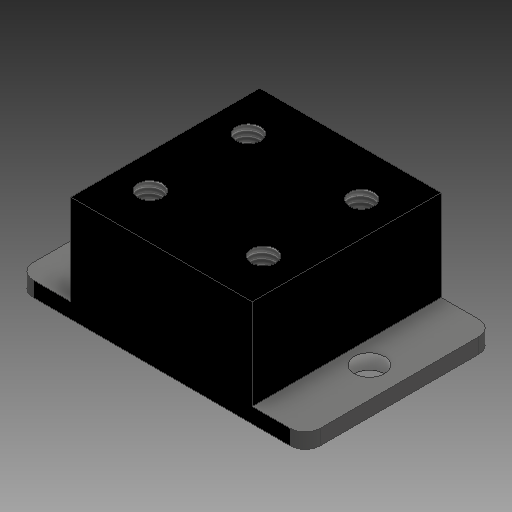
# Autodesk Inventor part: GT175DA120U
Saved by Autodesk Inventor 2019 (Build 230136000, 136)
## iProperties
Created: 2018-04-27
Part Number: GT175DA120U
Material: Generic
Document SubType Name: Modeling
Designer: Phil Erle
Density: 1 g/cm^3
Appearance: Default
Author: Phil Erle
Autodesk Inventor part; units mm, degrees
ref_plane "YZ Plane" through (0, 0, 0) normal (1, 0, 0) x (0, 1, 0)
ref_plane "XZ Plane" through (0, 0, 0) normal (0, 1, 0) x (-1, 0, 0)
ref_plane "XY Plane" through (0, 0, 0) normal (0, 0, 1) x (1, 0, 0)
sketch "Sketch1" plane through (0, 0, 0) normal (0, 0, 1) x (1, 0, 0)
  line L0 (-19, -12.5) -> (19, -12.5)
  line L1 (19, -12.5) -> (19, 12.5)
  line L2 (19, 12.5) -> (-19, 12.5)
  line L3 (-19, 12.5) -> (-19, -12.5)
  line L4 (-19, -12.5) -> (19, 12.5) construction
  line L5 (19, -12.5) -> (-19, 12.5) construction
  point P0 (0, 0)
  dimension "d0" = 38
  dimension "d1" = 25
  constraints: 12 end point, 2 midpoint, 2 parallel, 1 horizontal, 1 perpendicular
  measures "d0" distance of L1.end L2.end
  measures "d1" distance of L0.end L1.end
extrude "Extrusion1" add sketch "Sketch1" along normal blind 2
sketch "Sketch2" plane through (0, 0, 2) normal (0, 0, 1) x (1, 0, 0)
  line L0 (19, 12.5) -> (-19, 12.5) projected
  line L1 (-12, -12.5) -> (12, -12.5)
  line L2 (12, -12.5) -> (12, 12.5)
  line L3 (12, 12.5) -> (-12, 12.5)
  line L4 (-12, 12.5) -> (-12, -12.5)
  line L5 (-12, -12.5) -> (12, 12.5) construction
  line L6 (12, -12.5) -> (-12, 12.5) construction
  point P0 (0, 0)
  dimension "d4" = 24
  constraints: 12 end point, 2 midpoint, 2 parallel, 1 horizontal, 1 perpendicular, 1 point on line
  measures "d4" distance between parallel lines of L2 L4
extrude "Extrusion2" add sketch "Sketch2" along normal blind 12
sketch "Sketch3" plane through (0, 0, 2) normal (0, 0, 1) x (1, 0, 0)
  line L0 (-15, 0) -> (15, 0) construction
  point P0 (0, 0)
  point P1 (0, 0)
  dimension "d7" = 30
  constraints: 3 coincident, 2 end point, 1 horizontal, 1 horizontal alignment, 1 midpoint
  measures "d7" distance of L0.start L0.end
hole "Hole1" at (-15, 0, 2) at (15, 0, 2) direction (0, 0, -1) diameter 4 end through all
sketch "Sketch4" plane through (0, 0, 14) normal (0, 0, 1) x (1, 0, 0)
  line L0 (-7.5, -6.5) -> (7.5, -6.5) construction
  line L1 (7.5, -6.5) -> (7.5, 6.5) construction
  line L2 (7.5, 6.5) -> (-7.5, 6.5) construction
  line L3 (-7.5, 6.5) -> (-7.5, -6.5) construction
  line L4 (-7.5, -6.5) -> (7.5, 6.5) construction
  line L5 (7.5, -6.5) -> (-7.5, 6.5) construction
  point P0 (0, 0)
  dimension "d15" = 15
  dimension "d16" = 13
  constraints: 12 end point, 4 coincident, 2 midpoint, 2 parallel, 1 horizontal, 1 perpendicular
  measures "d15" distance of L1.end L2.end
  measures "d16" distance of L0.end L1.end
hole "Hole2" at (-7.5, 6.5, 14) at (7.5, 6.5, 14) at (7.5, -6.5, 14) at (-7.5, -6.5, 14) direction (0, 0, -1) diameter 3.242 depth 8 tip angle 118 thread size "M4x0.7" class "6H" standard "ISO Metric profile"
fillet "Fillet1" radius 2 4 edges at (-19, -12.5, 1) (19, -12.5, 1) (19, 12.5, 1) (-19, 12.5, 1)
body "Solid1"
